Autodesk Inventor part; units mm, degrees
(part 2 of 3)
  line L729 (108.7976, -134.2532) -> (108.7839, -134.2989)
  line L730 (108.7839, -134.2989) -> (108.7613, -134.3411)
  line L731 (108.7613, -134.3411) -> (108.7311, -134.3779)
  line L732 (108.7311, -134.3779) -> (108.694, -134.4084)
  line L733 (108.694, -134.4084) -> (108.6521, -134.4308)
  line L734 (108.6521, -134.4308) -> (108.6061, -134.4447)
  line L735 (108.6061, -134.4447) -> (108.5586, -134.4493)
  line L736 (108.5586, -134.4493) -> (107.6462, -134.4493)
  line L737 (107.6462, -134.4493) -> (107.5987, -134.4447)
  line L738 (107.5987, -134.4447) -> (107.5527, -134.4308)
  line L739 (107.5527, -134.4308) -> (107.5108, -134.4084)
  line L740 (107.5108, -134.4084) -> (107.4737, -134.3779)
  line L741 (107.4737, -134.3779) -> (107.4435, -134.3411)
  line L742 (107.4435, -134.3411) -> (107.4209, -134.2989)
  line L743 (107.4209, -134.2989) -> (107.4072, -134.2532)
  line L744 (107.4072, -134.2532) -> (107.4024, -134.2057)
  line L745 (107.4024, -134.2057) -> (107.4024, -133.718)
  line L746 (107.4024, -133.718) -> (107.4072, -133.6705)
  line L747 (107.4072, -133.6705) -> (107.4209, -133.6248)
  line L748 (107.4209, -133.6248) -> (107.4435, -133.5827)
  line L749 (107.4435, -133.5827) -> (107.4737, -133.5458)
  line L750 (107.4737, -133.5458) -> (107.5108, -133.5154)
  line L751 (107.5108, -133.5154) -> (107.5527, -133.493)
  line L752 (107.5527, -133.493) -> (107.5987, -133.479)
  line L753 (107.5987, -133.479) -> (107.6462, -133.4745)
  line L754 (107.6462, -133.4745) -> (108.5586, -133.4745)
  line L755 (108.5586, -133.4745) -> (108.6061, -133.479)
  line L756 (120.9759, -133.2504) -> (121.0219, -133.2644)
  line L757 (121.0219, -133.2644) -> (121.0638, -133.2868)
  line L758 (121.0638, -133.2868) -> (121.1009, -133.3172)
  line L759 (121.1009, -133.3172) -> (121.1311, -133.3541)
  line L760 (121.1311, -133.3541) -> (121.1537, -133.3962)
  line L761 (121.1537, -133.3962) -> (121.1674, -133.4419)
  line L762 (121.1674, -133.4419) -> (121.1722, -133.4894)
  line L763 (121.1722, -133.4894) -> (121.1722, -133.9771)
  line L764 (121.1722, -133.9771) -> (121.1674, -134.0246)
  line L765 (121.1674, -134.0246) -> (121.1537, -134.0703)
  line L766 (121.1537, -134.0703) -> (121.1311, -134.1125)
  line L767 (121.1311, -134.1125) -> (121.1009, -134.1493)
  line L768 (121.1009, -134.1493) -> (121.0638, -134.1798)
  line L769 (121.0638, -134.1798) -> (121.0219, -134.2022)
  line L770 (121.0219, -134.2022) -> (120.9759, -134.2161)
  line L771 (120.9759, -134.2161) -> (120.9284, -134.2207)
  line L772 (120.9284, -134.2207) -> (120.016, -134.2207)
  line L773 (120.016, -134.2207) -> (119.9685, -134.2161)
  line L774 (119.9685, -134.2161) -> (119.9225, -134.2022)
  line L775 (119.9225, -134.2022) -> (119.8806, -134.1798)
  line L776 (119.8806, -134.1798) -> (119.8436, -134.1493)
  line L777 (119.8436, -134.1493) -> (119.8133, -134.1125)
  line L778 (119.8133, -134.1125) -> (119.7907, -134.0703)
  line L779 (119.7907, -134.0703) -> (119.777, -134.0246)
  line L780 (119.777, -134.0246) -> (119.7722, -133.9771)
  line L781 (119.7722, -133.9771) -> (119.7722, -133.4894)
  line L782 (119.7722, -133.4894) -> (119.777, -133.4419)
  line L783 (119.777, -133.4419) -> (119.7907, -133.3962)
  line L784 (119.7907, -133.3962) -> (119.8133, -133.3541)
  line L785 (119.8133, -133.3541) -> (119.8436, -133.3172)
  line L786 (119.8436, -133.3172) -> (119.8806, -133.2868)
  line L787 (119.8806, -133.2868) -> (119.9225, -133.2644)
  line L788 (119.9225, -133.2644) -> (119.9685, -133.2504)
  line L789 (119.9685, -133.2504) -> (120.016, -133.2459)
  line L790 (120.016, -133.2459) -> (120.9284, -133.2459)
  line L791 (120.9284, -133.2459) -> (120.9759, -133.2504)
  line L792 (117.1791, -132.1895) -> (116.6292, -132.1895)
  line L793 (116.6292, -132.1895) -> (116.6292, -130.6893)
  line L794 (116.6292, -130.6893) -> (117.1791, -130.6893)
  line L795 (117.1791, -130.6893) -> (117.1791, -132.1895)
  line L796 (109.9792, -132.1895) -> (109.4293, -132.1895)
  line L797 (109.4293, -132.1895) -> (109.4293, -130.6893)
  line L798 (109.4293, -130.6893) -> (109.9792, -130.6893)
  line L799 (109.9792, -130.6893) -> (109.9792, -132.1895)
  line L800 (110.7793, -132.1895) -> (110.2291, -132.1895)
  line L801 (110.2291, -132.1895) -> (110.2291, -130.6893)
  line L802 (110.2291, -130.6893) -> (110.7793, -130.6893)
  line L803 (110.7793, -130.6893) -> (110.7793, -132.1895)
  line L804 (111.5792, -132.1895) -> (111.0292, -132.1895)
  line L805 (111.0292, -132.1895) -> (111.0292, -130.6893)
  line L806 (111.0292, -130.6893) -> (111.5792, -130.6893)
  line L807 (111.5792, -130.6893) -> (111.5792, -132.1895)
  line L808 (112.3793, -132.1895) -> (111.8291, -132.1895)
  line L809 (111.8291, -132.1895) -> (111.8291, -130.6893)
  line L810 (111.8291, -130.6893) -> (112.3793, -130.6893)
  line L811 (112.3793, -130.6893) -> (112.3793, -132.1895)
  line L812 (113.1791, -132.1895) -> (112.6292, -132.1895)
  line L813 (112.6292, -132.1895) -> (112.6292, -130.6893)
  line L814 (112.6292, -130.6893) -> (113.1791, -130.6893)
  line L815 (113.1791, -130.6893) -> (113.1791, -132.1895)
  line L816 (113.9792, -132.1895) -> (113.4293, -132.1895)
  line L817 (113.4293, -132.1895) -> (113.4293, -130.6893)
  line L818 (113.4293, -130.6893) -> (113.9792, -130.6893)
  line L819 (113.9792, -130.6893) -> (113.9792, -132.1895)
  line L820 (114.7793, -132.1895) -> (114.2291, -132.1895)
  line L821 (114.2291, -132.1895) -> (114.2291, -130.6893)
  line L822 (114.2291, -130.6893) -> (114.7793, -130.6893)
  line L823 (114.7793, -130.6893) -> (114.7793, -132.1895)
  line L824 (115.5791, -132.1895) -> (115.0292, -132.1895)
  line L825 (115.0292, -132.1895) -> (115.0292, -130.6893)
  line L826 (115.0292, -130.6893) -> (115.5791, -130.6893)
  line L827 (115.5791, -130.6893) -> (115.5791, -132.1895)
  line L828 (116.3792, -132.1895) -> (115.8291, -132.1895)
  line L829 (115.8291, -132.1895) -> (115.8291, -130.6893)
  line L830 (115.8291, -130.6893) -> (116.3792, -130.6893)
  line L831 (116.3792, -130.6893) -> (116.3792, -132.1895)
  line L832 (117.9792, -132.1895) -> (117.4293, -132.1895)
  line L833 (117.4293, -132.1895) -> (117.4293, -130.6893)
  line L834 (117.4293, -130.6893) -> (117.9792, -130.6893)
  line L835 (117.9792, -130.6893) -> (117.9792, -132.1895)
  line L836 (121.9779, -130.8941) -> (122.0236, -130.908)
  line L837 (122.0236, -130.908) -> (122.0658, -130.9304)
  line L838 (122.0658, -130.9304) -> (122.1029, -130.9609)
  line L839 (122.1029, -130.9609) -> (122.1331, -130.9977)
  line L840 (122.1331, -130.9977) -> (122.1557, -131.0399)
  line L841 (122.1557, -131.0399) -> (122.1694, -131.0856)
  line L842 (122.1694, -131.0856) -> (122.1743, -131.1331)
  line L843 (122.1743, -131.1331) -> (122.1743, -131.6208)
  line L844 (122.1743, -131.6208) -> (122.1694, -131.6683)
  line L845 (122.1694, -131.6683) -> (122.1557, -131.714)
  line L846 (122.1557, -131.714) -> (122.1331, -131.7561)
  line L847 (122.1331, -131.7561) -> (122.1029, -131.793)
  line L848 (122.1029, -131.793) -> (122.0658, -131.8232)
  line L849 (122.0658, -131.8232) -> (122.0236, -131.8458)
  line L850 (122.0236, -131.8458) -> (121.9779, -131.8598)
  line L851 (121.9779, -131.8598) -> (121.9304, -131.8644)
  line L852 (121.9304, -131.8644) -> (121.018, -131.8644)
  line L853 (121.018, -131.8644) -> (120.9703, -131.8598)
  line L854 (120.9703, -131.8598) -> (120.9246, -131.8458)
  line L855 (120.9246, -131.8458) -> (120.8824, -131.8232)
  line L856 (120.8824, -131.8232) -> (120.8456, -131.793)
  line L857 (120.8456, -131.793) -> (120.8154, -131.7561)
  line L858 (120.8154, -131.7561) -> (120.7927, -131.714)
  line L859 (120.7927, -131.714) -> (120.7788, -131.6683)
  line L860 (120.7788, -131.6683) -> (120.7742, -131.6208)
  line L861 (120.7742, -131.6208) -> (120.7742, -131.1331)
  line L862 (120.7742, -131.1331) -> (120.7788, -131.0856)
  line L863 (120.7788, -131.0856) -> (120.7927, -131.0399)
  line L864 (120.7927, -131.0399) -> (120.8154, -130.9977)
  line L865 (120.8154, -130.9977) -> (120.8456, -130.9609)
  line L866 (120.8456, -130.9609) -> (120.8824, -130.9304)
  line L867 (120.8824, -130.9304) -> (120.9246, -130.908)
  line L868 (120.9246, -130.908) -> (120.9703, -130.8941)
  line L869 (120.9703, -130.8941) -> (121.018, -130.8895)
  line L870 (121.018, -130.8895) -> (121.9304, -130.8895)
  line L871 (121.9304, -130.8895) -> (121.9779, -130.8941)
  line L872 (120.1542, -130.0145) -> (118.6543, -130.0145)
  line L873 (118.6543, -130.0145) -> (118.6543, -129.4643)
  line L874 (118.6543, -129.4643) -> (120.1542, -129.4643)
  line L875 (120.1542, -129.4643) -> (120.1542, -130.0145)
  line L876 (108.7542, -130.0145) -> (107.2543, -130.0145)
  line L877 (107.2543, -130.0145) -> (107.2543, -129.4643)
  line L878 (107.2543, -129.4643) -> (108.7542, -129.4643)
  line L879 (108.7542, -129.4643) -> (108.7542, -130.0145)
  line L880 (121.9779, -129.019) -> (122.0236, -129.033)
  line L881 (122.0236, -129.033) -> (122.0658, -129.0554)
  line L882 (122.0658, -129.0554) -> (122.1029, -129.0858)
  line L883 (122.1029, -129.0858) -> (122.1331, -129.1227)
  line L884 (122.1331, -129.1227) -> (122.1557, -129.1648)
  line L885 (122.1557, -129.1648) -> (122.1694, -129.2106)
  line L886 (122.1694, -129.2106) -> (122.1743, -129.2581)
  line L887 (122.1743, -129.2581) -> (122.1743, -129.7457)
  line L888 (122.1743, -129.7457) -> (122.1694, -129.7932)
  line L889 (122.1694, -129.7932) -> (122.1557, -129.839)
  line L890 (122.1557, -129.839) -> (122.1331, -129.8811)
  line L891 (122.1331, -129.8811) -> (122.1029, -129.918)
  line L892 (122.1029, -129.918) -> (122.0658, -129.9484)
  line L893 (122.0658, -129.9484) -> (122.0236, -129.9708)
  line L894 (122.0236, -129.9708) -> (121.9779, -129.9848)
  line L895 (121.9779, -129.9848) -> (121.9304, -129.9893)
  line L896 (121.9304, -129.9893) -> (121.018, -129.9893)
  line L897 (121.018, -129.9893) -> (120.9703, -129.9848)
  line L898 (120.9703, -129.9848) -> (120.9246, -129.9708)
  line L899 (120.9246, -129.9708) -> (120.8824, -129.9484)
  line L900 (120.8824, -129.9484) -> (120.8456, -129.918)
  line L901 (120.8456, -129.918) -> (120.8154, -129.8811)
  line L902 (120.8154, -129.8811) -> (120.7927, -129.839)
  line L903 (120.7927, -129.839) -> (120.7788, -129.7932)
  line L904 (120.7788, -129.7932) -> (120.7742, -129.7457)
  line L905 (120.7742, -129.7457) -> (120.7742, -129.2581)
  line L906 (120.7742, -129.2581) -> (120.7788, -129.2106)
  line L907 (120.7788, -129.2106) -> (120.7927, -129.1648)
  line L908 (120.7927, -129.1648) -> (120.8154, -129.1227)
  line L909 (120.8154, -129.1227) -> (120.8456, -129.0858)
  line L910 (120.8456, -129.0858) -> (120.8824, -129.0554)
  line L911 (120.8824, -129.0554) -> (120.9246, -129.033)
  line L912 (120.9246, -129.033) -> (120.9703, -129.019)
  line L913 (120.9703, -129.019) -> (121.018, -129.0145)
  line L914 (121.018, -129.0145) -> (121.9304, -129.0145)
  line L915 (121.9304, -129.0145) -> (121.9779, -129.019)
  line L916 (120.1542, -129.2144) -> (118.6543, -129.2144)
  line L917 (118.6543, -129.2144) -> (118.6543, -128.6645)
  line L918 (118.6543, -128.6645) -> (120.1542, -128.6645)
  line L919 (120.1542, -128.6645) -> (120.1542, -129.2144)
  line L920 (108.7542, -129.2144) -> (107.2543, -129.2144)
  line L921 (107.2543, -129.2144) -> (107.2543, -128.6645)
  line L922 (107.2543, -128.6645) -> (108.7542, -128.6645)
  line L923 (108.7542, -128.6645) -> (108.7542, -129.2144)
  line L924 (106.2693, -127.5563) -> (106.315, -127.5702)
  line L925 (106.315, -127.5702) -> (106.3572, -127.5926)
  line L926 (106.3572, -127.5926) -> (106.3942, -127.6231)
  line L927 (106.3942, -127.6231) -> (106.4245, -127.6599)
  line L928 (106.4245, -127.6599) -> (106.4471, -127.7021)
  line L929 (106.4471, -127.7021) -> (106.4608, -127.7478)
  line L930 (106.4608, -127.7478) -> (106.4656, -127.7953)
  line L931 (106.4656, -127.7953) -> (106.4656, -128.283)
  line L932 (106.4656, -128.283) -> (106.4608, -128.3305)
  line L933 (106.4608, -128.3305) -> (106.4471, -128.3762)
  line L934 (106.4471, -128.3762) -> (106.4245, -128.4183)
  line L935 (106.4245, -128.4183) -> (106.3942, -128.4552)
  line L936 (106.3942, -128.4552) -> (106.3572, -128.4856)
  line L937 (106.3572, -128.4856) -> (106.315, -128.508)
  line L938 (106.315, -128.508) -> (106.2693, -128.522)
  line L939 (106.2693, -128.522) -> (106.2218, -128.5265)
  line L940 (106.2218, -128.5265) -> (105.3094, -128.5265)
  line L941 (105.3094, -128.5265) -> (105.2619, -128.522)
  line L942 (105.2619, -128.522) -> (105.2159, -128.508)
  line L943 (105.2159, -128.508) -> (105.174, -128.4856)
  line L944 (105.174, -128.4856) -> (105.1369, -128.4552)
  line L945 (105.1369, -128.4552) -> (105.1067, -128.4183)
  line L946 (105.1067, -128.4183) -> (105.0841, -128.3762)
  line L947 (105.0841, -128.3762) -> (105.0704, -128.3305)
  line L948 (105.0704, -128.3305) -> (105.0656, -128.283)
  line L949 (105.0656, -128.283) -> (105.0656, -127.7953)
  line L950 (105.0656, -127.7953) -> (105.0704, -127.7478)
  line L951 (105.0704, -127.7478) -> (105.0841, -127.7021)
  line L952 (105.0841, -127.7021) -> (105.1067, -127.6599)
  line L953 (105.1067, -127.6599) -> (105.1369, -127.6231)
  line L954 (105.1369, -127.6231) -> (105.174, -127.5926)
  line L955 (105.174, -127.5926) -> (105.2159, -127.5702)
  line L956 (105.2159, -127.5702) -> (105.2619, -127.5563)
  line L957 (105.2619, -127.5563) -> (105.3094, -127.5517)
  line L958 (105.3094, -127.5517) -> (106.2218, -127.5517)
  line L959 (106.2218, -127.5517) -> (106.2693, -127.5563)
  line L960 (120.1542, -128.4145) -> (118.6543, -128.4145)
  line L961 (118.6543, -128.4145) -> (118.6543, -127.8644)
  line L962 (118.6543, -127.8644) -> (120.1542, -127.8644)
  line L963 (120.1542, -127.8644) -> (120.1542, -128.4145)
  line L964 (108.7542, -128.4145) -> (107.2543, -128.4145)
  line L965 (107.2543, -128.4145) -> (107.2543, -127.8644)
  line L966 (107.2543, -127.8644) -> (108.7542, -127.8644)
  line L967 (108.7542, -127.8644) -> (108.7542, -128.4145)
  line L968 (120.1542, -127.6144) -> (118.6543, -127.6144)
  line L969 (118.6543, -127.6144) -> (118.6543, -127.0645)
  line L970 (118.6543, -127.0645) -> (120.1542, -127.0645)
  line L971 (120.1542, -127.0645) -> (120.1542, -127.6144)
  line L972 (108.7542, -127.6144) -> (107.2543, -127.6144)
  line L973 (107.2543, -127.6144) -> (107.2543, -127.0645)
  line L974 (107.2543, -127.0645) -> (108.7542, -127.0645)
  line L975 (108.7542, -127.0645) -> (108.7542, -127.6144)
  line L976 (120.1542, -126.8143) -> (118.6543, -126.8143)
  line L977 (118.6543, -126.8143) -> (118.6543, -126.2644)
  line L978 (118.6543, -126.2644) -> (120.1542, -126.2644)
  line L979 (120.1542, -126.2644) -> (120.1542, -126.8143)
  line L980 (108.7542, -126.8143) -> (107.2543, -126.8143)
  line L981 (107.2543, -126.8143) -> (107.2543, -126.2644)
  line L982 (107.2543, -126.2644) -> (108.7542, -126.2644)
  line L983 (108.7542, -126.2644) -> (108.7542, -126.8143)
  line L984 (106.2693, -125.6812) -> (106.315, -125.6952)
  line L985 (106.315, -125.6952) -> (106.3572, -125.7176)
  line L986 (106.3572, -125.7176) -> (106.3942, -125.748)
  line L987 (106.3942, -125.748) -> (106.4245, -125.7849)
  line L988 (106.4245, -125.7849) -> (106.4471, -125.827)
  line L989 (106.4471, -125.827) -> (106.4608, -125.8727)
  line L990 (106.4608, -125.8727) -> (106.4656, -125.9202)
  line L991 (106.4656, -125.9202) -> (106.4656, -126.4079)
  line L992 (106.4656, -126.4079) -> (106.4608, -126.4554)
  line L993 (106.4608, -126.4554) -> (106.4471, -126.5011)
  line L994 (106.4471, -126.5011) -> (106.4245, -126.5433)
  line L995 (106.4245, -126.5433) -> (106.3942, -126.5801)
  line L996 (106.3942, -126.5801) -> (106.3572, -126.6106)
  line L997 (106.3572, -126.6106) -> (106.315, -126.633)
  line L998 (106.315, -126.633) -> (106.2693, -126.6469)
  line L999 (106.2693, -126.6469) -> (106.2218, -126.6515)
  line L1000 (106.2218, -126.6515) -> (105.3094, -126.6515)
  line L1001 (105.3094, -126.6515) -> (105.2619, -126.6469)
  line L1002 (105.2619, -126.6469) -> (105.2159, -126.633)
  line L1003 (105.2159, -126.633) -> (105.174, -126.6106)
  line L1004 (105.174, -126.6106) -> (105.1369, -126.5801)
  line L1005 (105.1369, -126.5801) -> (105.1067, -126.5433)
  line L1006 (105.1067, -126.5433) -> (105.0841, -126.5011)
  line L1007 (105.0841, -126.5011) -> (105.0704, -126.4554)
  line L1008 (105.0704, -126.4554) -> (105.0656, -126.4079)
  line L1009 (105.0656, -126.4079) -> (105.0656, -125.9202)
  line L1010 (105.0656, -125.9202) -> (105.0704, -125.8727)
  line L1011 (105.0704, -125.8727) -> (105.0841, -125.827)
  line L1012 (105.0841, -125.827) -> (105.1067, -125.7849)
  line L1013 (105.1067, -125.7849) -> (105.1369, -125.748)
  line L1014 (105.1369, -125.748) -> (105.174, -125.7176)
  line L1015 (105.174, -125.7176) -> (105.2159, -125.6952)
  line L1016 (105.2159, -125.6952) -> (105.2619, -125.6812)
  line L1017 (105.2619, -125.6812) -> (105.3094, -125.6767)
  line L1018 (105.3094, -125.6767) -> (106.2218, -125.6767)
  line L1019 (106.2218, -125.6767) -> (106.2693, -125.6812)
  line L1020 (120.1542, -126.0145) -> (118.6543, -126.0145)
  line L1021 (118.6543, -126.0145) -> (118.6543, -125.4643)
  line L1022 (118.6543, -125.4643) -> (120.1542, -125.4643)
  line L1023 (120.1542, -125.4643) -> (120.1542, -126.0145)
  line L1024 (108.7542, -126.0145) -> (107.2543, -126.0145)
  line L1025 (107.2543, -126.0145) -> (107.2543, -125.4643)
  line L1026 (107.2543, -125.4643) -> (108.7542, -125.4643)
  line L1027 (108.7542, -125.4643) -> (108.7542, -126.0145)
  line L1028 (120.1542, -125.2144) -> (118.6543, -125.2144)
  line L1029 (118.6543, -125.2144) -> (118.6543, -124.6645)
  line L1030 (118.6543, -124.6645) -> (120.1542, -124.6645)
  line L1031 (120.1542, -124.6645) -> (120.1542, -125.2144)
  line L1032 (108.7542, -125.2144) -> (107.2543, -125.2144)
  line L1033 (107.2543, -125.2144) -> (107.2543, -124.6645)
  line L1034 (107.2543, -124.6645) -> (108.7542, -124.6645)
  line L1035 (108.7542, -124.6645) -> (108.7542, -125.2144)
  line L1036 (106.2581, -124.1141) -> (106.3038, -124.128)
  line L1037 (106.3038, -124.128) -> (106.346, -124.1504)
  line L1038 (106.346, -124.1504) -> (106.3828, -124.1809)
  line L1039 (106.3828, -124.1809) -> (106.413, -124.2177)
  line L1040 (106.413, -124.2177) -> (106.4357, -124.2598)
  line L1041 (106.4357, -124.2598) -> (106.4496, -124.3056)
  line L1042 (106.4496, -124.3056) -> (106.4542, -124.3531)
  line L1043 (106.4542, -124.3531) -> (106.4542, -124.8407)
  line L1044 (106.4542, -124.8407) -> (106.4496, -124.8882)
  line L1045 (106.4496, -124.8882) -> (106.4357, -124.934)
  line L1046 (106.4357, -124.934) -> (106.413, -124.9761)
  line L1047 (106.413, -124.9761) -> (106.3828, -125.013)
  line L1048 (106.3828, -125.013) -> (106.346, -125.0434)
  line L1049 (106.346, -125.0434) -> (106.3038, -125.0658)
  line L1050 (106.3038, -125.0658) -> (106.2581, -125.0798)
  line L1051 (106.2581, -125.0798) -> (106.2104, -125.0843)
  line L1052 (106.2104, -125.0843) -> (105.298, -125.0843)
  line L1053 (105.298, -125.0843) -> (105.2505, -125.0798)
  line L1054 (105.2505, -125.0798) -> (105.2048, -125.0658)
  line L1055 (105.2048, -125.0658) -> (105.1626, -125.0434)
  line L1056 (105.1626, -125.0434) -> (105.1255, -125.013)
  line L1057 (105.1255, -125.013) -> (105.0953, -124.9761)
  line L1058 (105.0953, -124.9761) -> (105.0727, -124.934)
  line L1059 (105.0727, -124.934) -> (105.059, -124.8882)
  line L1060 (105.059, -124.8882) -> (105.0541, -124.8407)
  line L1061 (105.0541, -124.8407) -> (105.0541, -124.3531)
  line L1062 (105.0541, -124.3531) -> (105.059, -124.3056)
  line L1063 (105.059, -124.3056) -> (105.0727, -124.2598)
  line L1064 (105.0727, -124.2598) -> (105.0953, -124.2177)
  line L1065 (105.0953, -124.2177) -> (105.1255, -124.1809)
  line L1066 (105.1255, -124.1809) -> (105.1626, -124.1504)
  line L1067 (105.1626, -124.1504) -> (105.2048, -124.128)
  line L1068 (105.2048, -124.128) -> (105.2505, -124.1141)
  line L1069 (105.2505, -124.1141) -> (105.298, -124.1095)
  line L1070 (105.298, -124.1095) -> (106.2104, -124.1095)
  line L1071 (106.2104, -124.1095) -> (106.2581, -124.1141)
  line L1072 (120.1542, -124.4143) -> (118.6543, -124.4143)
  line L1073 (118.6543, -124.4143) -> (118.6543, -123.8644)
  line L1074 (118.6543, -123.8644) -> (120.1542, -123.8644)
  line L1075 (120.1542, -123.8644) -> (120.1542, -124.4143)
  line L1076 (108.7542, -124.4143) -> (107.2543, -124.4143)
  line L1077 (107.2543, -124.4143) -> (107.2543, -123.8644)
  line L1078 (107.2543, -123.8644) -> (108.7542, -123.8644)
  line L1079 (108.7542, -123.8644) -> (108.7542, -124.4143)
  line L1080 (120.1542, -123.6144) -> (118.6543, -123.6144)
  line L1081 (118.6543, -123.6144) -> (118.6543, -123.0645)
  line L1082 (118.6543, -123.0645) -> (120.1542, -123.0645)
  line L1083 (120.1542, -123.0645) -> (120.1542, -123.6144)
  line L1084 (108.7542, -123.6144) -> (107.2543, -123.6144)
  line L1085 (107.2543, -123.6144) -> (107.2543, -123.0645)
  line L1086 (107.2543, -123.0645) -> (108.7542, -123.0645)
  line L1087 (108.7542, -123.0645) -> (108.7542, -123.6144)
  line L1088 (106.2581, -122.239) -> (106.3038, -122.253)
  line L1089 (106.3038, -122.253) -> (106.346, -122.2756)
  line L1090 (106.346, -122.2756) -> (106.3828, -122.3058)
  line L1091 (106.3828, -122.3058) -> (106.413, -122.3427)
  line L1092 (106.413, -122.3427) -> (106.4357, -122.3848)
  line L1093 (106.4357, -122.3848) -> (106.4496, -122.4305)
  line L1094 (106.4496, -122.4305) -> (106.4542, -122.478)
  line L1095 (106.4542, -122.478) -> (106.4542, -122.9657)
  line L1096 (106.4542, -122.9657) -> (106.4496, -123.0132)
  line L1097 (106.4496, -123.0132) -> (106.4357, -123.0589)
  line L1098 (106.4357, -123.0589) -> (106.413, -123.1011)
  line L1099 (106.413, -123.1011) -> (106.3828, -123.1379)
  line L1100 (106.3828, -123.1379) -> (106.346, -123.1684)
  line L1101 (106.346, -123.1684) -> (106.3038, -123.1908)
  line L1102 (106.3038, -123.1908) -> (106.2581, -123.2047)
  line L1103 (106.2581, -123.2047) -> (106.2104, -123.2093)
  line L1104 (106.2104, -123.2093) -> (105.298, -123.2093)
  line L1105 (105.298, -123.2093) -> (105.2505, -123.2047)
  line L1106 (105.2505, -123.2047) -> (105.2048, -123.1908)
  line L1107 (105.2048, -123.1908) -> (105.1626, -123.1684)
  line L1108 (105.1626, -123.1684) -> (105.1255, -123.1379)
  line L1109 (105.1255, -123.1379) -> (105.0953, -123.1011)
  line L1110 (105.0953, -123.1011) -> (105.0727, -123.0589)
  line L1111 (105.0727, -123.0589) -> (105.059, -123.0132)
  line L1112 (105.059, -123.0132) -> (105.0541, -122.9657)
  line L1113 (105.0541, -122.9657) -> (105.0541, -122.478)
  line L1114 (105.0541, -122.478) -> (105.059, -122.4305)
  line L1115 (105.059, -122.4305) -> (105.0727, -122.3848)
  line L1116 (105.0727, -122.3848) -> (105.0953, -122.3427)
  line L1117 (105.0953, -122.3427) -> (105.1255, -122.3058)
  line L1118 (105.1255, -122.3058) -> (105.1626, -122.2756)
  line L1119 (105.1626, -122.2756) -> (105.2048, -122.253)
  line L1120 (105.2048, -122.253) -> (105.2505, -122.239)
  line L1121 (105.2505, -122.239) -> (105.298, -122.2345)
  line L1122 (105.298, -122.2345) -> (106.2104, -122.2345)
  line L1123 (106.2104, -122.2345) -> (106.2581, -122.239)
  line L1124 (120.1542, -122.8143) -> (118.6543, -122.8143)
  line L1125 (118.6543, -122.8143) -> (118.6543, -122.2644)
  line L1126 (118.6543, -122.2644) -> (120.1542, -122.2644)
  line L1127 (120.1542, -122.2644) -> (120.1542, -122.8143)
  line L1128 (108.7542, -122.8143) -> (107.2543, -122.8143)
  line L1129 (107.2543, -122.8143) -> (107.2543, -122.2644)
  line L1130 (107.2543, -122.2644) -> (108.7542, -122.2644)
  line L1131 (108.7542, -122.2644) -> (108.7542, -122.8143)
  line L1132 (120.1542, -122.0145) -> (118.6543, -122.0145)
  line L1133 (118.6543, -122.0145) -> (118.6543, -121.4643)
  line L1134 (118.6543, -121.4643) -> (120.1542, -121.4643)
  line L1135 (120.1542, -121.4643) -> (120.1542, -122.0145)
  line L1136 (108.7542, -122.0145) -> (107.2543, -122.0145)
  line L1137 (107.2543, -122.0145) -> (107.2543, -121.4643)
  line L1138 (107.2543, -121.4643) -> (108.7542, -121.4643)
  line L1139 (108.7542, -121.4643) -> (108.7542, -122.0145)
  line L1140 (122.1189, -120.9799) -> (122.1649, -120.9939)
  line L1141 (122.1649, -120.9939) -> (122.2068, -121.0163)
  line L1142 (122.2068, -121.0163) -> (122.2439, -121.0467)
  line L1143 (122.2439, -121.0467) -> (122.2741, -121.0836)
  line L1144 (122.2741, -121.0836) -> (122.2967, -121.1257)
  line L1145 (122.2967, -121.1257) -> (122.3104, -121.1715)
  line L1146 (122.3104, -121.1715) -> (122.3152, -121.219)
  line L1147 (122.3152, -121.219) -> (122.3152, -121.7066)
  line L1148 (122.3152, -121.7066) -> (122.3104, -121.7541)
  line L1149 (122.3104, -121.7541) -> (122.2967, -121.7999)
  line L1150 (122.2967, -121.7999) -> (122.2741, -121.842)
  line L1151 (122.2741, -121.842) -> (122.2439, -121.8789)
  line L1152 (122.2439, -121.8789) -> (122.2068, -121.9093)
  line L1153 (122.2068, -121.9093) -> (122.1649, -121.9317)
  line L1154 (122.1649, -121.9317) -> (122.1189, -121.9457)
  line L1155 (122.1189, -121.9457) -> (122.0714, -121.9502)
  line L1156 (122.0714, -121.9502) -> (121.159, -121.9502)
  line L1157 (121.159, -121.9502) -> (121.1115, -121.9457)
  line L1158 (121.1115, -121.9457) -> (121.0655, -121.9317)
  line L1159 (121.0655, -121.9317) -> (121.0236, -121.9093)
  line L1160 (121.0236, -121.9093) -> (120.9866, -121.8789)
  line L1161 (120.9866, -121.8789) -> (120.9563, -121.842)
  line L1162 (120.9563, -121.842) -> (120.9337, -121.7999)
  line L1163 (120.9337, -121.7999) -> (120.92, -121.7541)
  line L1164 (120.92, -121.7541) -> (120.9152, -121.7066)
  line L1165 (120.9152, -121.7066) -> (120.9152, -121.219)
  line L1166 (120.9152, -121.219) -> (120.92, -121.1715)
  line L1167 (120.92, -121.1715) -> (120.9337, -121.1257)
  line L1168 (120.9337, -121.1257) -> (120.9563, -121.0836)
  line L1169 (120.9563, -121.0836) -> (120.9866, -121.0467)
  line L1170 (120.9866, -121.0467) -> (121.0236, -121.0163)
  line L1171 (121.0236, -121.0163) -> (121.0655, -120.9939)
  line L1172 (121.0655, -120.9939) -> (121.1115, -120.9799)
  line L1173 (121.1115, -120.9799) -> (121.159, -120.9754)
  line L1174 (121.159, -120.9754) -> (122.0714, -120.9754)
  line L1175 (122.0714, -120.9754) -> (122.1189, -120.9799)
  line L1176 (109.9792, -120.7894) -> (109.4293, -120.7894)
  line L1177 (109.4293, -120.7894) -> (109.4293, -119.2893)
  line L1178 (109.4293, -119.2893) -> (109.9792, -119.2893)
  line L1179 (109.9792, -119.2893) -> (109.9792, -120.7894)
  line L1180 (110.7793, -120.7894) -> (110.2291, -120.7894)
  line L1181 (110.2291, -120.7894) -> (110.2291, -119.2893)
  line L1182 (110.2291, -119.2893) -> (110.7793, -119.2893)
  line L1183 (110.7793, -119.2893) -> (110.7793, -120.7894)
  line L1184 (111.5792, -120.7894) -> (111.0292, -120.7894)
  line L1185 (111.0292, -120.7894) -> (111.0292, -119.2893)
  line L1186 (111.0292, -119.2893) -> (111.5792, -119.2893)
  line L1187 (111.5792, -119.2893) -> (111.5792, -120.7894)
  line L1188 (113.1791, -120.7894) -> (112.6292, -120.7894)
  line L1189 (112.6292, -120.7894) -> (112.6292, -119.2893)
  line L1190 (112.6292, -119.2893) -> (113.1791, -119.2893)
  line L1191 (113.1791, -119.2893) -> (113.1791, -120.7894)
  line L1192 (117.9792, -120.7894) -> (117.4293, -120.7894)
  line L1193 (117.4293, -120.7894) -> (117.4293, -119.2893)
  line L1194 (117.4293, -119.2893) -> (117.9792, -119.2893)
  line L1195 (117.9792, -119.2893) -> (117.9792, -120.7894)
  line L1196 (117.1791, -120.7894) -> (116.6292, -120.7894)
  line L1197 (116.6292, -120.7894) -> (116.6292, -119.2893)
  line L1198 (116.6292, -119.2893) -> (117.1791, -119.2893)
  line L1199 (117.1791, -119.2893) -> (117.1791, -120.7894)
  line L1200 (116.3792, -120.7894) -> (115.8291, -120.7894)
  line L1201 (115.8291, -120.7894) -> (115.8291, -119.2893)
  line L1202 (115.8291, -119.2893) -> (116.3792, -119.2893)
  line L1203 (116.3792, -119.2893) -> (116.3792, -120.7894)
  line L1204 (115.5791, -120.7894) -> (115.0292, -120.7894)
  line L1205 (115.0292, -120.7894) -> (115.0292, -119.2893)
  line L1206 (115.0292, -119.2893) -> (115.5791, -119.2893)
  line L1207 (115.5791, -119.2893) -> (115.5791, -120.7894)
  line L1208 (114.7793, -120.7894) -> (114.2291, -120.7894)
  line L1209 (114.2291, -120.7894) -> (114.2291, -119.2893)
  line L1210 (114.2291, -119.2893) -> (114.7793, -119.2893)
  line L1211 (114.7793, -119.2893) -> (114.7793, -120.7894)
  line L1212 (112.3793, -120.7894) -> (111.8291, -120.7894)
  line L1213 (111.8291, -120.7894) -> (111.8291, -119.2893)
  line L1214 (111.8291, -119.2893) -> (112.3793, -119.2893)
  line L1215 (112.3793, -119.2893) -> (112.3793, -120.7894)
  line L1216 (113.9792, -120.7894) -> (113.4293, -120.7894)
  line L1217 (113.4293, -120.7894) -> (113.4293, -119.2893)
  line L1218 (113.4293, -119.2893) -> (113.9792, -119.2893)
  line L1219 (113.9792, -119.2893) -> (113.9792, -120.7894)
  line L1220 (122.1189, -119.1049) -> (122.1649, -119.1189)
  line L1221 (122.1649, -119.1189) -> (122.2068, -119.1415)
  line L1222 (122.2068, -119.1415) -> (122.2439, -119.1717)
  line L1223 (122.2439, -119.1717) -> (122.2741, -119.2086)
  line L1224 (122.2741, -119.2086) -> (122.2967, -119.2507)
  line L1225 (122.2967, -119.2507) -> (122.3104, -119.2964)
  line L1226 (122.3104, -119.2964) -> (122.3152, -119.3439)
  line L1227 (122.3152, -119.3439) -> (122.3152, -119.8316)
  line L1228 (122.3152, -119.8316) -> (122.3104, -119.8791)
  line L1229 (122.3104, -119.8791) -> (122.2967, -119.9248)
  line L1230 (122.2967, -119.9248) -> (122.2741, -119.967)
  line L1231 (122.2741, -119.967) -> (122.2439, -120.0038)
  line L1232 (122.2439, -120.0038) -> (122.2068, -120.0343)
  line L1233 (122.2068, -120.0343) -> (122.1649, -120.0567)
  line L1234 (122.1649, -120.0567) -> (122.1189, -120.0706)
  line L1235 (122.1189, -120.0706) -> (122.0714, -120.0752)
  line L1236 (122.0714, -120.0752) -> (121.159, -120.0752)
  line L1237 (121.159, -120.0752) -> (121.1115, -120.0706)
  line L1238 (121.1115, -120.0706) -> (121.0655, -120.0567)
  line L1239 (121.0655, -120.0567) -> (121.0236, -120.0343)
  line L1240 (121.0236, -120.0343) -> (120.9866, -120.0038)
  line L1241 (120.9866, -120.0038) -> (120.9563, -119.967)
  line L1242 (120.9563, -119.967) -> (120.9337, -119.9248)
  line L1243 (120.9337, -119.9248) -> (120.92, -119.8791)
  line L1244 (120.92, -119.8791) -> (120.9152, -119.8316)
  line L1245 (120.9152, -119.8316) -> (120.9152, -119.3439)
  line L1246 (120.9152, -119.3439) -> (120.92, -119.2964)
  line L1247 (120.92, -119.2964) -> (120.9337, -119.2507)
  line L1248 (120.9337, -119.2507) -> (120.9563, -119.2086)
  line L1249 (120.9563, -119.2086) -> (120.9866, -119.1717)
  line L1250 (120.9866, -119.1717) -> (121.0236, -119.1415)
  line L1251 (121.0236, -119.1415) -> (121.0655, -119.1189)
  line L1252 (121.0655, -119.1189) -> (121.1115, -119.1049)
  line L1253 (121.1115, -119.1049) -> (121.159, -119.1003)
  line L1254 (121.159, -119.1003) -> (122.0714, -119.1003)
  line L1255 (122.0714, -119.1003) -> (122.1189, -119.1049)
  line L1256 (119.9805, -117.094) -> (120.0262, -117.108)
  line L1257 (120.0262, -117.108) -> (120.0683, -117.1306)
  line L1258 (120.0683, -117.1306) -> (120.1054, -117.1608)
  line L1259 (120.1054, -117.1608) -> (120.1356, -117.1976)
  line L1260 (120.1356, -117.1976) -> (120.1583, -117.2398)
  line L1261 (120.1583, -117.2398) -> (120.172, -117.2855)
  line L1262 (120.172, -117.2855) -> (120.1768, -117.3333)
  line L1263 (120.1768, -117.3333) -> (120.1768, -118.2456)
  line L1264 (120.1768, -118.2456) -> (120.172, -118.2931)
  line L1265 (120.172, -118.2931) -> (120.1583, -118.3389)
  line L1266 (120.1583, -118.3389) -> (120.1356, -118.381)
  line L1267 (120.1356, -118.381) -> (120.1054, -118.4181)
  line L1268 (120.1054, -118.4181) -> (120.0683, -118.4483)
  line L1269 (120.0683, -118.4483) -> (120.0262, -118.4709)
  line L1270 (120.0262, -118.4709) -> (119.9805, -118.4846)
  line L1271 (119.9805, -118.4846) -> (119.933, -118.4895)
  line L1272 (119.933, -118.4895) -> (119.4455, -118.4895)
  line L1273 (119.4455, -118.4895) -> (119.3978, -118.4846)
  line L1274 (119.3978, -118.4846) -> (119.3521, -118.4709)
  line L1275 (119.3521, -118.4709) -> (119.3102, -118.4483)
  line L1276 (119.3102, -118.4483) -> (119.2731, -118.4181)
  line L1277 (119.2731, -118.4181) -> (119.2428, -118.381)
  line L1278 (119.2428, -118.381) -> (119.2202, -118.3389)
  line L1279 (119.2202, -118.3389) -> (119.2063, -118.2931)
  line L1280 (119.2063, -118.2931) -> (119.2017, -118.2456)
  line L1281 (119.2017, -118.2456) -> (119.2017, -117.3333)
  line L1282 (119.2017, -117.3333) -> (119.2063, -117.2855)
  line L1283 (119.2063, -117.2855) -> (119.2202, -117.2398)
  line L1284 (119.2202, -117.2398) -> (119.2428, -117.1976)
  line L1285 (119.2428, -117.1976) -> (119.2731, -117.1608)
  line L1286 (119.2731, -117.1608) -> (119.3102, -117.1306)
  line L1287 (119.3102, -117.1306) -> (119.3521, -117.108)
  line L1288 (119.3521, -117.108) -> (119.3978, -117.094)
  line L1289 (119.3978, -117.094) -> (119.4455, -117.0894)
  line L1290 (119.4455, -117.0894) -> (119.933, -117.0894)
  line L1291 (119.933, -117.0894) -> (119.9805, -117.094)
  line L1292 (118.1054, -117.094) -> (118.1511, -117.108)
  line L1293 (118.1511, -117.108) -> (118.1933, -117.1306)
  line L1294 (118.1933, -117.1306) -> (118.2304, -117.1608)
  line L1295 (118.2304, -117.1608) -> (118.2606, -117.1976)
  line L1296 (118.2606, -117.1976) -> (118.2832, -117.2398)
  line L1297 (118.2832, -117.2398) -> (118.2969, -117.2855)
  line L1298 (118.2969, -117.2855) -> (118.3018, -117.3333)
  line L1299 (118.3018, -117.3333) -> (118.3018, -118.2456)
  line L1300 (118.3018, -118.2456) -> (118.2969, -118.2931)
  line L1301 (118.2969, -118.2931) -> (118.2832, -118.3389)
  line L1302 (118.2832, -118.3389) -> (118.2606, -118.381)
  line L1303 (118.2606, -118.381) -> (118.2304, -118.4181)
  line L1304 (118.2304, -118.4181) -> (118.1933, -118.4483)
  line L1305 (118.1933, -118.4483) -> (118.1511, -118.4709)
  line L1306 (118.1511, -118.4709) -> (118.1054, -118.4846)
  line L1307 (118.1054, -118.4846) -> (118.0579, -118.4895)
  line L1308 (118.0579, -118.4895) -> (117.5705, -118.4895)
  line L1309 (117.5705, -118.4895) -> (117.523, -118.4846)
  line L1310 (117.523, -118.4846) -> (117.4773, -118.4709)
  line L1311 (117.4773, -118.4709) -> (117.4351, -118.4483)
  line L1312 (117.4351, -118.4483) -> (117.398, -118.4181)
  line L1313 (117.398, -118.4181) -> (117.3678, -118.381)
  line L1314 (117.3678, -118.381) -> (117.3452, -118.3389)
  line L1315 (117.3452, -118.3389) -> (117.3315, -118.2931)
  line L1316 (117.3315, -118.2931) -> (117.3267, -118.2456)
  line L1317 (117.3267, -118.2456) -> (117.3267, -117.3333)
  line L1318 (117.3267, -117.3333) -> (117.3315, -117.2855)
  line L1319 (117.3315, -117.2855) -> (117.3452, -117.2398)
  line L1320 (117.3452, -117.2398) -> (117.3678, -117.1976)
  line L1321 (117.3678, -117.1976) -> (117.398, -117.1608)
  line L1322 (117.398, -117.1608) -> (117.4351, -117.1306)
  line L1323 (117.4351, -117.1306) -> (117.4773, -117.108)
  line L1324 (117.4773, -117.108) -> (117.523, -117.094)
  line L1325 (117.523, -117.094) -> (117.5705, -117.0894)
  line L1326 (117.5705, -117.0894) -> (118.0579, -117.0894)
  line L1327 (118.0579, -117.0894) -> (118.1054, -117.094)
  line L1328 (108.0379, -117.0541) -> (108.0836, -117.0678)
  line L1329 (108.0836, -117.0678) -> (108.1258, -117.0904)
  line L1330 (108.1258, -117.0904) -> (108.1629, -117.1207)
  line L1331 (108.1629, -117.1207) -> (108.1931, -117.1578)
  line L1332 (108.1931, -117.1578) -> (108.2157, -117.1999)
  line L1333 (108.2157, -117.1999) -> (108.2294, -117.2456)
  line L1334 (108.2294, -117.2456) -> (108.2342, -117.2931)
  line L1335 (108.2342, -117.2931) -> (108.2342, -118.2058)
  line L1336 (108.2342, -118.2058) -> (108.2294, -118.2533)
  line L1337 (108.2294, -118.2533) -> (108.2157, -118.299)
  line L1338 (108.2157, -118.299) -> (108.1931, -118.3411)
  line L1339 (108.1931, -118.3411) -> (108.1629, -118.378)
  line L1340 (108.1629, -118.378) -> (108.1258, -118.4082)
  line L1341 (108.1258, -118.4082) -> (108.0836, -118.4308)
  line L1342 (108.0836, -118.4308) -> (108.0379, -118.4448)
  line L1343 (108.0379, -118.4448) -> (107.9904, -118.4493)
  line L1344 (107.9904, -118.4493) -> (107.503, -118.4493)
  line L1345 (107.503, -118.4493) -> (107.4555, -118.4448)
  line L1346 (107.4555, -118.4448) -> (107.4097, -118.4308)
  line L1347 (107.4097, -118.4308) -> (107.3676, -118.4082)
  line L1348 (107.3676, -118.4082) -> (107.3305, -118.378)
  line L1349 (107.3305, -118.378) -> (107.3003, -118.3411)
  line L1350 (107.3003, -118.3411) -> (107.2777, -118.299)
  line L1351 (107.2777, -118.299) -> (107.2639, -118.2533)
  line L1352 (107.2639, -118.2533) -> (107.2591, -118.2058)
  line L1353 (107.2591, -118.2058) -> (107.2591, -117.2931)
  line L1354 (107.2591, -117.2931) -> (107.2639, -117.2456)
  line L1355 (107.2639, -117.2456) -> (107.2777, -117.1999)
  line L1356 (107.2777, -117.1999) -> (107.3003, -117.1578)
  line L1357 (107.3003, -117.1578) -> (107.3305, -117.1207)
  line L1358 (107.3305, -117.1207) -> (107.3676, -117.0904)
  line L1359 (107.3676, -117.0904) -> (107.4097, -117.0678)
  line L1360 (107.4097, -117.0678) -> (107.4555, -117.0541)
  line L1361 (107.4555, -117.0541) -> (107.503, -117.0493)
  line L1362 (107.503, -117.0493) -> (107.9904, -117.0493)
  line L1363 (107.9904, -117.0493) -> (108.0379, -117.0541)
  line L1364 (109.9129, -117.0541) -> (109.9586, -117.0678)
  line L1365 (109.9586, -117.0678) -> (110.0008, -117.0904)
  line L1366 (110.0008, -117.0904) -> (110.0379, -117.1207)
  line L1367 (110.0379, -117.1207) -> (110.0681, -117.1578)
  line L1368 (110.0681, -117.1578) -> (110.0907, -117.1999)
  line L1369 (110.0907, -117.1999) -> (110.1044, -117.2456)
  line L1370 (110.1044, -117.2456) -> (110.1093, -117.2931)
  line L1371 (110.1093, -117.2931) -> (110.1093, -118.2058)
  line L1372 (110.1093, -118.2058) -> (110.1044, -118.2533)
  line L1373 (110.1044, -118.2533) -> (110.0907, -118.299)
  line L1374 (110.0907, -118.299) -> (110.0681, -118.3411)
  line L1375 (110.0681, -118.3411) -> (110.0379, -118.378)
  line L1376 (110.0379, -118.378) -> (110.0008, -118.4082)
  line L1377 (110.0008, -118.4082) -> (109.9586, -118.4308)
  line L1378 (109.9586, -118.4308) -> (109.9129, -118.4448)
  line L1379 (109.9129, -118.4448) -> (109.8654, -118.4493)
  line L1380 (109.8654, -118.4493) -> (109.378, -118.4493)
  line L1381 (109.378, -118.4493) -> (109.3305, -118.4448)
  line L1382 (109.3305, -118.4448) -> (109.2848, -118.4308)
  line L1383 (109.2848, -118.4308) -> (109.2426, -118.4082)
  line L1384 (109.2426, -118.4082) -> (109.2055, -118.378)
  line L1385 (109.2055, -118.378) -> (109.1753, -118.3411)
  line L1386 (109.1753, -118.3411) -> (109.1527, -118.299)
  line L1387 (109.1527, -118.299) -> (109.139, -118.2533)
  line L1388 (109.139, -118.2533) -> (109.1341, -118.2058)
  line L1389 (109.1341, -118.2058) -> (109.1341, -117.2931)
  line L1390 (109.1341, -117.2931) -> (109.139, -117.2456)
  line L1391 (109.139, -117.2456) -> (109.1527, -117.1999)
  line L1392 (109.1527, -117.1999) -> (109.1753, -117.1578)
  line L1393 (109.1753, -117.1578) -> (109.2055, -117.1207)
  line L1394 (109.2055, -117.1207) -> (109.2426, -117.0904)
  line L1395 (109.2426, -117.0904) -> (109.2848, -117.0678)
  line L1396 (109.2848, -117.0678) -> (109.3305, -117.0541)
  line L1397 (109.3305, -117.0541) -> (109.378, -117.0493)
  line L1398 (109.378, -117.0493) -> (109.8654, -117.0493)
  line L1399 (109.8654, -117.0493) -> (109.9129, -117.0541)
  line L1400 (134.2644, -118.237) -> (133.7056, -118.237)
  line L1401 (133.7056, -118.237) -> (133.7056, -116.7765)
  line L1402 (133.7056, -116.7765) -> (134.2644, -116.7765)
  line L1403 (134.2644, -116.7765) -> (134.2644, -118.237)
  line L1404 (132.9944, -118.237) -> (132.4356, -118.237)
  line L1405 (132.4356, -118.237) -> (132.4356, -116.7765)
  line L1406 (132.4356, -116.7765) -> (132.9944, -116.7765)
  line L1407 (132.9944, -116.7765) -> (132.9944, -118.237)
  line L1408 (129.1844, -118.237) -> (128.6256, -118.237)
  line L1409 (128.6256, -118.237) -> (128.6256, -116.7765)
  line L1410 (128.6256, -116.7765) -> (129.1844, -116.7765)
  line L1411 (129.1844, -116.7765) -> (129.1844, -118.237)
  line L1412 (127.9144, -118.237) -> (127.3556, -118.237)
  line L1413 (127.3556, -118.237) -> (127.3556, -116.7765)
  line L1414 (127.3556, -116.7765) -> (127.9144, -116.7765)
  line L1415 (127.9144, -116.7765) -> (127.9144, -118.237)
  line L1416 (131.7244, -118.237) -> (131.1656, -118.237)
  line L1417 (131.1656, -118.237) -> (131.1656, -116.7765)
  line L1418 (131.1656, -116.7765) -> (131.7244, -116.7765)
  line L1419 (131.7244, -116.7765) -> (131.7244, -118.237)
  line L1420 (130.4544, -118.237) -> (129.8956, -118.237)
  line L1421 (129.8956, -118.237) -> (129.8956, -116.7765)
  line L1422 (129.8956, -116.7765) -> (130.4544, -116.7765)
  line L1423 (130.4544, -116.7765) -> (130.4544, -118.237)
  line L1424 (126.6444, -118.237) -> (126.0856, -118.237)
  line L1425 (126.0856, -118.237) -> (126.0856, -116.7765)
  line L1426 (126.0856, -116.7765) -> (126.6444, -116.7765)
  line L1427 (126.6444, -116.7765) -> (126.6444, -118.237)
  line L1428 (124.7351, -114.9325) -> (124.7808, -114.9464)
  line L1429 (124.7808, -114.9464) -> (124.823, -114.9688)
  line L1430 (124.823, -114.9688) -> (124.8601, -114.9993)
  line L1431 (124.8601, -114.9993) -> (124.8903, -115.0361)
  line L1432 (124.8903, -115.0361) -> (124.9129, -115.0783)
  line L1433 (124.9129, -115.0783) -> (124.9266, -115.124)
  line L1434 (124.9266, -115.124) -> (124.9314, -115.1715)
  line L1435 (124.9314, -115.1715) -> (124.9314, -115.6592)
  line L1436 (124.9314, -115.6592) -> (124.9266, -115.7067)
  line L1437 (124.9266, -115.7067) -> (124.9129, -115.7524)
  line L1438 (124.9129, -115.7524) -> (124.8903, -115.7945)
  line L1439 (124.8903, -115.7945) -> (124.8601, -115.8314)
  line L1440 (124.8601, -115.8314) -> (124.823, -115.8618)
  line L1441 (124.823, -115.8618) -> (124.7808, -115.8842)
  line L1442 (124.7808, -115.8842) -> (124.7351, -115.8982)
  line L1443 (124.7351, -115.8982) -> (124.6876, -115.9027)
  line L1444 (124.6876, -115.9027) -> (123.7752, -115.9027)
  line L1445 (123.7752, -115.9027) -> (123.7277, -115.8982)
  line L1446 (123.7277, -115.8982) -> (123.682, -115.8842)
  line L1447 (123.682, -115.8842) -> (123.6398, -115.8618)
  line L1448 (123.6398, -115.8618) -> (123.6028, -115.8314)
  line L1449 (123.6028, -115.8314) -> (123.5725, -115.7945)
  line L1450 (123.5725, -115.7945) -> (123.5499, -115.7524)
  line L1451 (123.5499, -115.7524) -> (123.5362, -115.7067)
  line L1452 (123.5362, -115.7067) -> (123.5314, -115.6592)
  line L1453 (123.5314, -115.6592) -> (123.5314, -115.1715)
  line L1454 (123.5314, -115.1715) -> (123.5362, -115.124)
  line L1455 (123.5362, -115.124) -> (123.5499, -115.0783)
  line L1456 (123.5499, -115.0783) -> (123.5725, -115.0361)
  line L1457 (123.5725, -115.0361) -> (123.6028, -114.9993)
  line L1458 (123.6028, -114.9993) -> (123.6398, -114.9688)
  line L1459 (123.6398, -114.9688) -> (123.682, -114.9464)
  line L1460 (123.682, -114.9464) -> (123.7277, -114.9325)
  line L1461 (123.7277, -114.9325) -> (123.7752, -114.9279)
  line L1462 (123.7752, -114.9279) -> (124.6876, -114.9279)
  line L1463 (124.6876, -114.9279) -> (124.7351, -114.9325)
  line L1464 (96.1741, -113.3762) -> (96.2198, -113.3899)
  line L1465 (96.2198, -113.3899) -> (96.2619, -113.4125)
  line L1466 (96.2619, -113.4125) -> (96.2988, -113.4427)
  line L1467 (96.2988, -113.4427) -> (96.3292, -113.4798)
  line L1468 (96.3292, -113.4798) -> (96.3516, -113.5217)
  line L1469 (96.3516, -113.5217) -> (96.3656, -113.5677)
  line L1470 (96.3656, -113.5677) -> (96.3701, -113.6152)
  line L1471 (96.3701, -113.6152) -> (96.3701, -114.5276)
  line L1472 (96.3701, -114.5276) -> (96.3656, -114.5751)
  line L1473 (96.3656, -114.5751) -> (96.3516, -114.6208)
  line L1474 (96.3516, -114.6208) -> (96.3292, -114.663)
  line L1475 (96.3292, -114.663) -> (96.2988, -114.7)
  line L1476 (96.2988, -114.7) -> (96.2619, -114.7303)
  line L1477 (96.2619, -114.7303) -> (96.2198, -114.7529)
  line L1478 (96.2198, -114.7529) -> (96.1741, -114.7666)
  line L1479 (96.1741, -114.7666) -> (96.1266, -114.7714)
  line L1480 (96.1266, -114.7714) -> (95.6389, -114.7714)
  line L1481 (95.6389, -114.7714) -> (95.5914, -114.7666)
  line L1482 (95.5914, -114.7666) -> (95.5457, -114.7529)
  line L1483 (95.5457, -114.7529) -> (95.5035, -114.7303)
  line L1484 (95.5035, -114.7303) -> (95.4667, -114.7)
  line L1485 (95.4667, -114.7) -> (95.4362, -114.663)
  line L1486 (95.4362, -114.663) -> (95.4138, -114.6208)
  line L1487 (95.4138, -114.6208) -> (95.3999, -114.5751)
  line L1488 (95.3999, -114.5751) -> (95.3953, -114.5276)
  line L1489 (95.3953, -114.5276) -> (95.3953, -113.6152)
  line L1490 (95.3953, -113.6152) -> (95.3999, -113.5677)
  line L1491 (95.3999, -113.5677) -> (95.4138, -113.5217)
  line L1492 (95.4138, -113.5217) -> (95.4362, -113.4798)
  line L1493 (95.4362, -113.4798) -> (95.4667, -113.4427)
  line L1494 (95.4667, -113.4427) -> (95.5035, -113.4125)
  line L1495 (95.5035, -113.4125) -> (95.5457, -113.3899)
  line L1496 (95.5457, -113.3899) -> (95.5914, -113.3762)
  line L1497 (95.5914, -113.3762) -> (95.6389, -113.3714)
  line L1498 (95.6389, -113.3714) -> (96.1266, -113.3714)
  line L1499 (96.1266, -113.3714) -> (96.1741, -113.3762)
  line L1500 (94.299, -113.3762) -> (94.3447, -113.3899)
  line L1501 (94.3447, -113.3899) -> (94.3869, -113.4125)
  line L1502 (94.3869, -113.4125) -> (94.4237, -113.4427)
  line L1503 (94.4237, -113.4427) -> (94.4542, -113.4798)
  line L1504 (94.4542, -113.4798) -> (94.4766, -113.5217)
  line L1505 (94.4766, -113.5217) -> (94.4905, -113.5677)
  line L1506 (94.4905, -113.5677) -> (94.4951, -113.6152)
  line L1507 (94.4951, -113.6152) -> (94.4951, -114.5276)
  line L1508 (94.4951, -114.5276) -> (94.4905, -114.5751)
  line L1509 (94.4905, -114.5751) -> (94.4766, -114.6208)
  line L1510 (94.4766, -114.6208) -> (94.4542, -114.663)
  line L1511 (94.4542, -114.663) -> (94.4237, -114.7)
  line L1512 (94.4237, -114.7) -> (94.3869, -114.7303)
  line L1513 (94.3869, -114.7303) -> (94.3447, -114.7529)
  line L1514 (94.3447, -114.7529) -> (94.299, -114.7666)
  line L1515 (94.299, -114.7666) -> (94.2515, -114.7714)
  line L1516 (94.2515, -114.7714) -> (93.7638, -114.7714)
  line L1517 (93.7638, -114.7714) -> (93.7163, -114.7666)
  line L1518 (93.7163, -114.7666) -> (93.6706, -114.7529)
  line L1519 (93.6706, -114.7529) -> (93.6285, -114.7303)
  line L1520 (93.6285, -114.7303) -> (93.5916, -114.7)
  line L1521 (93.5916, -114.7) -> (93.5612, -114.663)
  line L1522 (93.5612, -114.663) -> (93.5388, -114.6208)
  line L1523 (93.5388, -114.6208) -> (93.5248, -114.5751)
  line L1524 (93.5248, -114.5751) -> (93.5203, -114.5276)
  line L1525 (93.5203, -114.5276) -> (93.5203, -113.6152)
  line L1526 (93.5203, -113.6152) -> (93.5248, -113.5677)
  line L1527 (93.5248, -113.5677) -> (93.5388, -113.5217)
  line L1528 (93.5388, -113.5217) -> (93.5612, -113.4798)
  line L1529 (93.5612, -113.4798) -> (93.5916, -113.4427)
  line L1530 (93.5916, -113.4427) -> (93.6285, -113.4125)
  line L1531 (93.6285, -113.4125) -> (93.6706, -113.3899)
  line L1532 (93.6706, -113.3899) -> (93.7163, -113.3762)
  line L1533 (93.7163, -113.3762) -> (93.7638, -113.3714)
  line L1534 (93.7638, -113.3714) -> (94.2515, -113.3714)
  line L1535 (94.2515, -113.3714) -> (94.299, -113.3762)
  line L1536 (124.7351, -113.0574) -> (124.7808, -113.0714)
  line L1537 (124.7808, -113.0714) -> (124.823, -113.0938)
  line L1538 (124.823, -113.0938) -> (124.8601, -113.1242)
  line L1539 (124.8601, -113.1242) -> (124.8903, -113.1611)
  line L1540 (124.8903, -113.1611) -> (124.9129, -113.2032)
  line L1541 (124.9129, -113.2032) -> (124.9266, -113.2489)
  line L1542 (124.9266, -113.2489) -> (124.9314, -113.2964)
  line L1543 (124.9314, -113.2964) -> (124.9314, -113.7841)
  line L1544 (124.9314, -113.7841) -> (124.9266, -113.8316)
  line L1545 (124.9266, -113.8316) -> (124.9129, -113.8773)
  line L1546 (124.9129, -113.8773) -> (124.8903, -113.9195)
  line L1547 (124.8903, -113.9195) -> (124.8601, -113.9563)
  line L1548 (124.8601, -113.9563) -> (124.823, -113.9868)
  line L1549 (124.823, -113.9868) -> (124.7808, -114.0092)
  line L1550 (124.7808, -114.0092) -> (124.7351, -114.0231)
  line L1551 (124.7351, -114.0231) -> (124.6876, -114.0277)
  line L1552 (124.6876, -114.0277) -> (123.7752, -114.0277)
  line L1553 (123.7752, -114.0277) -> (123.7277, -114.0231)
  line L1554 (123.7277, -114.0231) -> (123.682, -114.0092)
  line L1555 (123.682, -114.0092) -> (123.6398, -113.9868)
  line L1556 (123.6398, -113.9868) -> (123.6028, -113.9563)
  line L1557 (123.6028, -113.9563) -> (123.5725, -113.9195)
  line L1558 (123.5725, -113.9195) -> (123.5499, -113.8773)
  line L1559 (123.5499, -113.8773) -> (123.5362, -113.8316)
  line L1560 (123.5362, -113.8316) -> (123.5314, -113.7841)
  line L1561 (123.5314, -113.7841) -> (123.5314, -113.2964)
  line L1562 (123.5314, -113.2964) -> (123.5362, -113.2489)
  line L1563 (123.5362, -113.2489) -> (123.5499, -113.2032)
  line L1564 (123.5499, -113.2032) -> (123.5725, -113.1611)
  line L1565 (123.5725, -113.1611) -> (123.6028, -113.1242)
  line L1566 (123.6028, -113.1242) -> (123.6398, -113.0938)
  line L1567 (123.6398, -113.0938) -> (123.682, -113.0714)
  line L1568 (123.682, -113.0714) -> (123.7277, -113.0574)
  line L1569 (123.7277, -113.0574) -> (123.7752, -113.0529)
  line L1570 (123.7752, -113.0529) -> (124.6876, -113.0529)
  line L1571 (124.6876, -113.0529) -> (124.7351, -113.0574)
  line L1572 (126.6444, -112.7887) -> (126.0856, -112.7887)